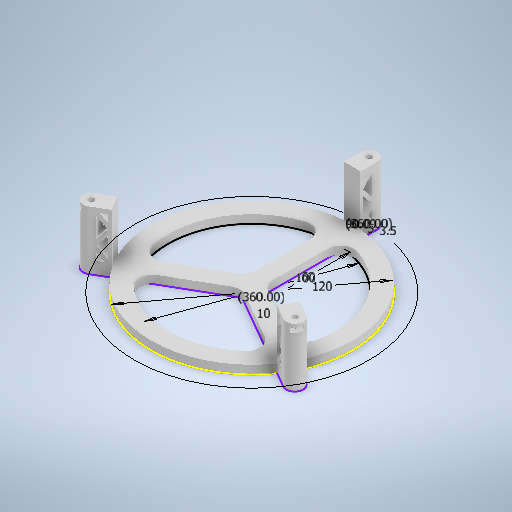
# Autodesk Inventor part: Bottom_Stand
Saved by Autodesk Inventor 2025.1 (Build 291241000, 241)
## iProperties
Created: 2026-04-16
Part Number: Bottom_Stand
Material: Generic
Document SubType Name: Modeling
Designer: ryand
Density: 1 g/cm^3
Appearance: Default
Author: ryand
Autodesk Inventor part; units mm, degrees
ref_plane "YZ Plane" through (0, 0, 0) normal (1, 0, 0) x (0, 1, 0)
ref_plane "XZ Plane" through (0, 0, 0) normal (0, 1, 0) x (-1, 0, 0)
ref_plane "XY Plane" through (0, 0, 0) normal (0, 0, 1) x (1, 0, 0)
sketch "Sketch1" plane through (0, 0, 0) normal (0, 1, 0) x (-1, 0, 0)
  circle A0 centre (0, 0) radius 60
  circle A1 centre (0, 0) radius 50
  circle A2 centre (0, 0) radius 5
  line L0 (5, 0) -> (-5, 0)
  line L1 (-5, 0) -> (-5, -50)
  line L2 (-5, -50) -> (5, -50)
  line L3 (5, -50) -> (5, 0)
  line L4 (2.5, -4.3301) -> (45.8013, 20.6699)
  line L5 (40.8013, 29.3301) -> (-2.5, 4.3301)
  line L6 (2.5, 4.3301) -> (-40.8013, 29.3301)
  line L7 (-45.8013, 20.6699) -> (-2.5, -4.3301)
  point P0 (0, 5.7735)
  point P1 (-40.5842, 29.2048)
  point P2 (40.5842, 29.2048)
  point P3 (5, -2.8868)
  point P4 (45.5842, 20.5446)
  point P5 (5, -49.7494)
  point P6 (-5, -2.8868)
  point P7 (-5, -49.7494)
  point P8 (-45.5842, 20.5446)
  dimension "d2" = 10
  dimension "d0" = 120
  dimension "d1" = 100
  dimension "d3" = 50
  dimension "d6" = 360
  constraints: 16 end point, 3 coincident, 2 centre point, 2 parallel, 1 horizontal, 1 horizontal alignment, 1 perpendicular, 21 other
  measures "d0" diameter of A0
  measures "d1" diameter of A1
  measures "d3" distance of L1.end L0.end
extrude "Extrusion1" add sketch "Sketch1" along normal blind 5 contours A0 | L4 L3 A2 L6 L5 A1 | L3 L2 A1 | A1 L1 L7 A2 L4 L3 | L4 A2 L3 | L2 L1 A1 | L6 L5 A2 L1 L7 A1 | L6 A2 L5 | L0 A2 | A2 L0 | A2 L7 L1
sketch "Sketch3" plane through (0, 0, 0) normal (0, -1, 0) x (1, 0, 0)
  circle A0 centre (0, -70) radius 1.75
  arc A1 (-5, -70) -> (5, -70) centre (0, -70) ccw
  line L0 (-5, -70) -> (-5, -59.7913)
  circle A2 centre (0, 0) radius 60 projected
  line L1 (-5, -70) -> (5.2087, -70) construction
  line L2 (5, -70) -> (5, -59.7913)
  arc A3 (-5, -59.7913) -> (5, -59.7913) centre (0, 0) ccw
  circle A4 centre (60.6218, 35) radius 1.75
  line L3 (63.1218, 30.6699) -> (58.0174, 39.5109) construction
  arc A5 (63.1218, 30.6699) -> (58.1218, 39.3301) centre (60.6218, 35) ccw
  line L4 (58.1218, 39.3301) -> (49.2808, 34.2258)
  line L5 (63.1218, 30.6699) -> (54.2808, 25.5655)
  arc A6 (54.2808, 25.5655) -> (49.2808, 34.2258) centre (0, 0) ccw
  circle A7 centre (-60.6218, 35) radius 1.75
  line L6 (-58.1218, 39.3301) -> (-63.2261, 30.4891) construction
  arc A8 (-58.1218, 39.3301) -> (-63.1218, 30.6699) centre (-60.6218, 35) ccw
  line L7 (-63.1218, 30.6699) -> (-54.2808, 25.5655)
  line L8 (-58.1218, 39.3301) -> (-49.2808, 34.2258)
  arc A9 (-49.2808, 34.2258) -> (-54.2808, 25.5655) centre (0, 0) ccw
  dimension "d10" = 3.5
  dimension "d12" = 5
  dimension "d21" = 90
  dimension "d24" = 360
  constraints: 18 end point, 14 point on circle, 9 centre point, 4 coincident, 1 horizontal, 1 perpendicular, 43 other
  measures "d10" diameter of A0
  measures "d12" distance of L2.start A0.centre
  measures "d21" angle of L1 L0
extrude "Extrusion3" add sketch "Sketch3" against normal blind 35 contours L0 A2 L2 A1 | L7 A8 L8 A2 | A2 L4 A5 L5
sketch "Sketch4" plane through (58.1218, 0, 39.3301) normal (-0.5, 0, 0.8660254) x (0.8660254, 0, 0.5)
  line L0 (0, 0) -> (0, 35) projected
  line L1 (-10.2087, 5) -> (-10.2087, 35) projected
  line L2 (-10.2087, 5) -> (-95.5655, 5) projected
  line L3 (-10.2087, 35) -> (0, 35) projected
  line L4 (-8.4587, 32.5) -> (-3.4587, 32.5)
  line L5 (-3.4587, 32.5) -> (-3.4587, 7.5)
  line L6 (-3.4587, 7.5) -> (-8.4587, 7.5)
  line L7 (-8.4587, 7.5) -> (-8.4587, 32.5)
  line L8 (-8.4587, 7.5) -> (-1.3876, 7.5) construction
  line L9 (-8.4587, 7.5) -> (1.5413, 7.5) construction
  line L10 (-9.3247, 8) -> (-7.3247, 8) construction
  line L11 (-8.4587, 7.5) -> (-0.6801, 7.5) construction
  line L12 (-3.4587, 13.581) -> (-3.4587, 17.081)
  line L13 (-3.4587, 17.081) -> (4.3199, 17.081) construction
  line L14 (-8.4587, 22.919) -> (-8.4587, 26.419)
  line L15 (-8.4587, 26.419) -> (-8.4587, 24.669)
  line L16 (-8.4587, 24.669) -> (-3.4587, 30.75)
  line L17 (-8.4587, 26.419) -> (-8.4587, 28.169)
  line L18 (-8.4587, 28.169) -> (-4.8976, 32.5)
  line L19 (-8.4587, 24.669) -> (-3.4587, 18.831)
  line L20 (-8.4587, 22.919) -> (-8.4587, 21.169)
  line L21 (-8.4587, 21.169) -> (-3.4587, 15.331)
  line L22 (-8.4587, 7.5) -> (-8.4587, 9.25)
  line L23 (-8.4587, 9.25) -> (-3.4587, 15.331)
  line L24 (-3.4587, 13.581) -> (-3.4587, 11.831)
  line L25 (-3.4587, 11.831) -> (-7.0198, 7.5)
  point P0 (-70, 0)
  point P1 (-7.0198, 7.5)
  dimension "d28" = 10.2087
  dimension "d29" = 30
  dimension "d30" = 5
  dimension "d31" = 25
  dimension "d32" = 2.5
  dimension "d33" = 1.75
  dimension "d66" = 3.5
  dimension "d69" = 3.5
  dimension "d70" = 1.75
  dimension "d71" = 1.75
  dimension "d72" = 1.75
  dimension "d73" = 1.75
  dimension "d74" = 1.75
  dimension "d118" = 1.75
  constraints: 44 end point, 11 point on line, 6 horizontal, 6 parallel, 2 midpoint, 1 collinear, 1 perpendicular
  measures "d28" distance between parallel lines of L0 L1
  measures "d29" distance between parallel lines of L2 L3
  measures "d30" distance of L5.end L6.end
  measures "d31" distance of L4.end L5.end
  measures "d32" distance between parallel lines of L3 L4
  measures "d33" distance between parallel lines of L1 L7
  measures "d66" distance of L12.start L12.end
  measures "d69" distance of L14.start L14.end
  measures "d70" distance of L14.end L15.end
  measures "d71" distance of L14.end L17.end
  measures "d72" distance of L14.start L20.end
  measures "d73" distance of L6.end L22.end
  measures "d74" distance of L12.start L24.end
  measures "d118" distance of L4.end L16.end
extrude "Extrusion4" cut sketch "Sketch4" against normal blind 10 contours L4 L18 L7 | L5 L19 L16 | L21 L23 L7 | L5 L6 L25
sketch "Sketch5" plane through (-63.1218, 0, 30.6699) normal (-0.5, 0, -0.8660254) x (-0.8660254, 0, 0.5)
  line L0 (-9.9161, 4.9711) -> (-63.7395, 4.9711)
  line L1 (-8.4587, 32.4711) -> (-3.4587, 32.4711)
  line L2 (-3.4587, 32.4711) -> (-3.4587, 7.4711)
  line L3 (-3.4587, 7.4711) -> (-8.4587, 7.4711)
  line L4 (-8.4587, 7.4711) -> (-8.4587, 32.4711)
  line L5 (-8.4587, 7.4711) -> (-1.3876, 7.4711) construction
  line L6 (-8.4587, 7.4711) -> (1.5413, 7.4711) construction
  line L7 (-9.0321, 7.9711) -> (-7.0321, 7.9711) construction
  line L8 (-8.4587, 7.4711) -> (-0.6801, 7.4711) construction
  line L9 (-3.4587, 13.5535) -> (-3.4587, 17.0535)
  line L10 (-3.4587, 17.0535) -> (4.3199, 17.0535) construction
  line L11 (-8.4587, 22.8886) -> (-8.4587, 26.3886)
  line L12 (-8.4587, 26.3886) -> (-8.4587, 24.6386)
  line L13 (-8.4587, 24.6386) -> (-3.4587, 30.7211)
  line L14 (-8.4587, 26.3886) -> (-8.4587, 28.1386)
  line L15 (-8.4587, 28.1386) -> (-4.8973, 32.4711)
  line L16 (-8.4587, 24.6386) -> (-3.4587, 18.8035)
  line L17 (-8.4587, 22.8886) -> (-8.4587, 21.1386)
  line L18 (-8.4587, 21.1386) -> (-3.4587, 15.3035)
  line L19 (-8.4587, 7.4711) -> (-8.4587, 9.2211)
  line L20 (-8.4587, 9.2211) -> (-3.4587, 15.3035)
  line L21 (-3.4587, 13.5535) -> (-3.4587, 11.8035)
  line L22 (-3.4587, 11.8035) -> (-7.0201, 7.4711)
  line L23 (-10.2087, 5) -> (-10.2087, 35) projected
  point P0 (-70, 0)
  point P1 (-38.174, 4.7574)
  point P2 (24.8357, 12.2574)
  point P3 (-8.4587, 24.6386)
  dimension "d85" = 5
  dimension "d86" = 25
  dimension "d89" = 3.5
  dimension "d90" = 3.5
  dimension "d91" = 1.75
  dimension "d92" = 1.75
  dimension "d93" = 1.75
  dimension "d94" = 1.75
  dimension "d95" = 1.75
  dimension "d96" = 1.75
  dimension "d97" = 2.5
  dimension "d119" = 1.75
  constraints: 46 end point, 11 point on line, 6 horizontal, 6 parallel, 3 midpoint, 1 perpendicular
  measures "d85" distance of L2.end L3.end
  measures "d86" distance of L1.end L2.end
  measures "d89" distance of L9.start L9.end
  measures "d90" distance of L11.start L11.end
  measures "d91" distance of L11.end L12.end
  measures "d92" distance of L11.end L14.end
  measures "d93" distance of L11.start L17.end
  measures "d94" distance of L3.end L19.end
  measures "d95" distance of L9.start L21.end
  measures "d96" distance from line of L23 point (-8.459, 24.639)
  measures "d97" distance from line of L0 L22.end
  measures "d119" distance of L1.end L13.end
extrude "Extrusion5" cut sketch "Sketch5" against normal blind 10 contours L1 L15 L4 | L2 L16 L13 | L18 L20 L4 | L2 L3 L22
sketch "Sketch6" plane through (5, 0, -59.7913) normal (1, 0, 0) x (0, 0, -1)
  line L0 (0.041, 4.7496) -> (-60.3749, 4.7496)
  line L1 (1.75, 32.5) -> (6.75, 32.5)
  line L2 (6.75, 32.5) -> (6.75, 7.5)
  line L3 (6.75, 7.5) -> (1.75, 7.5)
  line L4 (1.75, 7.5) -> (1.75, 32.5)
  line L5 (1.75, 7.5) -> (8.8211, 7.5) construction
  line L6 (1.75, 7.5) -> (11.75, 7.5) construction
  line L7 (0.925, 7.7496) -> (2.925, 7.7496) construction
  line L8 (1.75, 7.5) -> (9.5286, 7.5) construction
  line L9 (6.75, 13.4588) -> (6.75, 16.9588)
  line L10 (6.75, 16.9588) -> (14.5286, 16.9588) construction
  line L11 (1.75, 23.0412) -> (1.75, 26.5412)
  line L12 (1.75, 26.5412) -> (1.75, 24.7912)
  line L13 (1.75, 24.7912) -> (6.75, 30.75)
  line L14 (1.75, 26.5412) -> (1.75, 28.2912)
  line L15 (1.75, 28.2912) -> (5.2816, 32.5)
  line L16 (1.75, 24.7912) -> (6.75, 18.7088)
  line L17 (1.75, 23.0412) -> (1.75, 21.2912)
  line L18 (1.75, 21.2912) -> (6.75, 15.2088)
  line L19 (1.75, 7.5) -> (1.75, 9.25)
  line L20 (1.75, 9.25) -> (6.75, 15.2088)
  line L21 (6.75, 13.4588) -> (6.75, 11.7088)
  line L22 (0, 5) -> (0, 35) projected
  line L23 (0, 5) -> (-85.3568, 5) projected
  line L24 (0, 35) -> (10.2087, 35) projected
  line L25 (6.75, 11.7088) -> (3.2184, 7.5)
  line L26 (6.75, 11.7088) -> (12.2442, 11.7088) construction
  point P0 (-59.7913, 0)
  point P1 (-34.8094, 2.7365)
  point P2 (28.2003, 10.2365)
  point P3 (1.75, 24.7912)
  point P4 (4.25, 7.5)
  point P5 (3.2184, 7.5)
  dimension "d102" = 5
  dimension "d103" = 25
  dimension "d106" = 3.5
  dimension "d107" = 3.5
  dimension "d108" = 1.75
  dimension "d109" = 1.75
  dimension "d110" = 1.75
  dimension "d111" = 1.75
  dimension "d112" = 1.75
  dimension "d113" = 1.75
  dimension "d116" = 2.5
  dimension "d117" = 1.75
  dimension "d121" = 130
  dimension "d122" = 1.75
  constraints: 48 end point, 11 point on line, 7 horizontal, 6 parallel, 4 midpoint, 1 equal length, 1 perpendicular
  measures "d102" distance of L2.end L3.end
  measures "d103" distance of L1.end L2.end
  measures "d106" distance of L9.start L9.end
  measures "d107" distance of L11.start L11.end
  measures "d108" distance of L11.end L12.end
  measures "d109" distance of L11.end L14.end
  measures "d110" distance of L11.start L17.end
  measures "d111" distance of L3.end L19.end
  measures "d112" distance of L9.start L21.end
  measures "d113" distance from line of L22 point (1.75, 24.791)
  measures "d116" distance from line of L24 L15.end
  measures "d117" distance of L1.end L13.end
  measures "d121" angle of L25 L26
  measures "d122" distance of L9.end L16.end
extrude "Extrusion6" cut sketch "Sketch6" against normal blind 10 contours L1 L15 L4 | L2 L16 L13 | L18 L20 L4 | L2 L3 L25
ref_plane "Work Plane1" through (64.9519, 0, 37.5) normal (0.8660254, 0, 0.5) x (0.5, 0, -0.8660254)
sketch "Sketch7" plane through (64.9519, 0, 37.5) normal (0.8660254, 0, 0.5) x (0.5, 0, -0.8660254)
  line L0 (-3.1, 33) -> (3.1, 33)
  line L1 (3.1, 33) -> (3.1, 30.3)
  line L2 (3.1, 30.3) -> (-3.1, 30.3)
  line L3 (-3.1, 30.3) -> (-3.1, 33)
  line L4 (5, 35) -> (-5, 35) projected
  line L5 (-5, 0) -> (-5, 35) projected
  point P0 (0, 0)
  dimension "d125" = 6.2
  dimension "d126" = 2.7
  dimension "d127" = 2
  dimension "d128" = 1.9
  constraints: 8 end point, 2 parallel, 1 horizontal, 1 perpendicular
  measures "d125" distance of L1.end L2.end
  measures "d126" distance of L0.end L1.end
  measures "d127" distance between parallel lines of L4 L0
  measures "d128" distance between parallel lines of L5 L3
extrude "Extrusion7" cut sketch "Sketch7" against normal blind 8.1
ref_plane "Work Plane2" through (0, 0, -75) normal (0, 0, -1) x (-1, 0, 0)
sketch "Sketch8" plane through (0, 0, -75) normal (0, 0, -1) x (-1, 0, 0)
  line L0 (-3.1, 33) -> (3.1, 33)
  line L1 (3.1, 33) -> (3.1, 30.3)
  line L2 (3.1, 30.3) -> (-3.1, 30.3)
  line L3 (-3.1, 30.3) -> (-3.1, 33)
  line L4 (-5, 0) -> (-5, 35) projected
  line L5 (5, 35) -> (-5, 35) projected
  point P0 (0, 0)
  dimension "d131" = 6.2
  dimension "d132" = 2.7
  dimension "d133" = 1.9
  dimension "d134" = 2
  constraints: 8 end point, 2 parallel, 1 horizontal, 1 perpendicular
  measures "d131" distance of L1.end L2.end
  measures "d132" distance of L0.end L1.end
  measures "d133" distance between parallel lines of L4 L3
  measures "d134" distance between parallel lines of L5 L0
extrude "Extrusion8" cut sketch "Sketch8" against normal blind 8.1
ref_plane "Work Plane3" through (-64.9519, 0, 37.5) normal (-0.8660254, 0, 0.5) x (0.5, 0, 0.8660254)
sketch "Sketch9" plane through (-64.9519, 0, 37.5) normal (-0.8660254, 0, 0.5) x (0.5, 0, 0.8660254)
  line L0 (-3.1, 33) -> (3.1, 33)
  line L1 (3.1, 33) -> (3.1, 30.3)
  line L2 (3.1, 30.3) -> (-3.1, 30.3)
  line L3 (-3.1, 30.3) -> (-3.1, 33)
  line L4 (5, 35) -> (-5, 35) projected
  line L5 (-5, 0) -> (-5, 35) projected
  point P0 (0, 0)
  point P1 (0, 35)
  dimension "d137" = 6.2
  dimension "d138" = 2.7
  dimension "d139" = 2
  dimension "d140" = 1.9
  constraints: 8 end point, 2 parallel, 1 horizontal, 1 midpoint, 1 perpendicular
  measures "d137" distance of L1.end L2.end
  measures "d138" distance of L0.end L1.end
  measures "d139" distance from line of point (0, 35) L0
  measures "d140" distance between parallel lines of L5 L3
extrude "Extrusion9" cut sketch "Sketch9" against normal blind 8.1
fillet "Fillet1" radius 8 9 edges at (-5, 2.5, -49.7494) (5, 2.5, -49.7494) (45.5842, 2.5, 20.5446) (40.5842, 2.5, 29.2048) (-40.5842, 2.5, 29.2048) (-45.5842, 2.5, 20.5446) (-5, 2.5, -2.8868) (0, 2.5, 5.7735) (5, 2.5, -2.8868)
body "Solid1"
